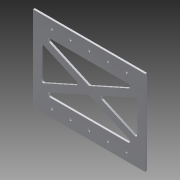
# Autodesk Inventor part: cross_structural_plate(csp)
Saved by Autodesk Inventor 2015 (Build 190159000, 159)
## iProperties
Created: 2015-11-03
Part Number: cross_structural_plate(csp)
Material: Aluminum 6061
Document SubType Name: Sheet Metal
Designer: elilitwack
Density: 2.7 g/cm^3
Sheet Metal Rule: Default
Appearance: Aluminum - Flat
Mass: 129.421 g
Surface Area: 365.561 cm^2
Volume: 47.9336 cm^3
Author: elilitwack
Autodesk Inventor part; units mm, degrees
ref_plane "YZ Plane" through (0, 0, 0) normal (1, 0, 0) x (0, 1, 0)
ref_plane "XZ Plane" through (0, 0, 0) normal (0, 1, 0) x (-1, 0, 0)
ref_plane "XY Plane" through (0, 0, 0) normal (0, 0, 1) x (1, 0, 0)
sketch "profile sketch" plane through (0, 0, 0) normal (0, 0, 1) x (1, 0, 0)
  line L0 (0, 0) -> (180.34, 0)
  line L1 (180.34, 0) -> (180.34, 136.5504)
  line L2 (180.34, 136.5504) -> (0, 136.5504)
  line L3 (0, 136.5504) -> (0, 0)
  dimension "d5" = 180.34
  dimension "d6" = 136.5504
  measures "d5" distance of L1.end L2.end
  measures "d6" distance of L0.end L1.end
extrude "Plate1" add sketch "profile sketch" along normal blind 3.048
sketch "rv_hole_sketch" plane through (0, 0, 3.048) normal (0, 0, 1) x (1, 0, 0)
  line L0 (0, 136.5504) -> (0, 0) construction
  line L1 (180.34, 0) -> (180.34, 136.5504) construction
  line L2 (0, 136.5504) -> (180.34, 136.5504) construction
  line L3 (180.34, 0) -> (0, 0) construction
  line L4 (0, 123.8504) -> (30.0567, 123.8504) construction
  line L5 (30.0567, 123.8504) -> (60.1133, 123.8504) construction
  line L6 (60.1133, 123.8504) -> (90.17, 123.8504) construction
  line L7 (90.17, 123.8504) -> (120.2267, 123.8504) construction
  line L8 (120.2267, 123.8504) -> (150.2833, 123.8504) construction
  line L9 (150.2833, 123.8504) -> (180.34, 123.8504) construction
  line L10 (0, 12.7) -> (30.0567, 12.7) construction
  line L11 (30.0567, 12.7) -> (60.1133, 12.7) construction
  line L12 (60.1133, 12.7) -> (90.17, 12.7) construction
  line L13 (90.17, 12.7) -> (120.2267, 12.7) construction
  line L14 (120.2267, 12.7) -> (150.2833, 12.7) construction
  line L15 (150.2833, 12.7) -> (180.34, 12.7) construction
  dimension "d10" = 12.7
  dimension "d11" = 12.7
  constraints: 24 end point, 13 point on line, 10 coincident, 10 collinear, 3 horizontal
  measures "d10" distance between parallel lines of L3 L13
  measures "d11" distance between parallel lines of L2 L6
hole "rv_holes" at (30.0567, 123.8504, 3.048) at (60.1133, 123.8504, 3.048) at (90.17, 123.8504, 3.048) at (120.2267, 123.8504, 3.048) at (150.2833, 123.8504, 3.048) at (150.2833, 12.7, 3.048) at (120.2267, 12.7, 3.048) at (90.17, 12.7, 3.048) at (60.1133, 12.7, 3.048) at (30.0567, 12.7, 3.048) direction (0, 0, -1) diameter 3.5719 depth 3.048 tip angle 118
sketch "cutout_sketch" plane through (0, 0, 3.048) normal (0, 0, 1) x (1, 0, 0)
  line L0 (12.7, 109.3645) -> (90.17, 74.6252)
  line L1 (90.17, 74.6252) -> (167.64, 109.3645)
  line L2 (167.64, 109.3645) -> (12.7, 109.3645)
  line L3 (12.7, 27.1859) -> (90.17, 61.9252)
  line L4 (90.17, 61.9252) -> (167.64, 27.1859)
  line L5 (167.64, 27.1859) -> (12.7, 27.1859)
  circle A0 centre (90.17, 123.8504) radius 1.7859 projected
  circle A1 centre (90.17, 12.7) radius 1.7859 projected
  line L6 (0, 0) -> (0, 136.5504) projected
  line L7 (180.34, 136.5504) -> (180.34, 0) projected
  line L8 (90.17, 74.6252) -> (90.17, 61.9252) construction
  line L9 (12.7, 96.6645) -> (76.0092, 68.2752)
  line L10 (76.0092, 68.2752) -> (12.7, 39.8859)
  line L11 (12.7, 39.8859) -> (12.7, 96.6645)
  line L12 (167.64, 96.6645) -> (104.3308, 68.2752)
  line L13 (104.3308, 68.2752) -> (167.64, 39.8859)
  line L14 (167.64, 39.8859) -> (167.64, 96.6645)
  line L15 (167.64, 109.3645) -> (167.64, 27.1859) construction
  line L16 (12.7, 109.3645) -> (12.7, 27.1859) construction
  dimension "d36" = 12.7
  dimension "d37" = 12.7
  dimension "d38" = 12.7
  dimension "d39" = 12.7
  dimension "d40" = 12.7
  dimension "d41" = 12.7
  dimension "d42" = 12.7
  dimension "d43" = 12.7
  constraints: 30 end point, 6 equal length, 5 parallel, 3 vertical, 2 collinear, 2 horizontal
  measures "d36" distance edge to line of A0 L2
  measures "d37" distance edge to line of A1 L5
  measures "d38" distance of L0.end L3.end
  measures "d39" distance from line of L6 L3.start
  measures "d40" distance from line of L7 L4.end
  measures "d41" distance of L0.start L9.start
  measures "d42" distance of L3.start L10.end
  measures "d43" distance of L1.end L12.start
extrude "Cut2" cut sketch "cutout_sketch" against normal blind 3.048 contours L2 L1 L0 | L3 L4 L5 | L9 L10 L11 | L14 L13 L12
fillet "Corner Round3" radius 3.175 12 edges at (12.7, 109.3645, 1.524) (167.64, 109.3645, 1.524) (90.17, 74.6252, 1.524) (12.7, 39.8859, 1.524) (12.7, 96.6645, 1.524) (76.0092, 68.2752, 1.524) (90.17, 61.9252, 1.524) (12.7, 27.1859, 1.524) (167.64, 27.1859, 1.524) (104.3308, 68.2752, 1.524) (167.64, 96.6645, 1.524) (167.64, 39.8859, 1.524)
equation "\"d5\" = bh_length"
equation "\"d6\" = bp_height"
equation "\"d10\" = 0.5 * cb_outer_diameter"
equation "\"d11\" = 0.5 * cb_outer_diameter"
equation "\"d12\" = rv_hole_diameter"
equation "\"d17\" = Thickness"
equation "\"d36\" = cmp_mounting_margins"
equation "\"d37\" = cmp_mounting_margins"
equation "\"d38\" = cmp_mounting_margins"
equation "\"d39\" = cmp_mounting_margins"
equation "\"d40\" = cmp_mounting_margins"
equation "\"d41\" = cmp_mounting_margins"
equation "\"d42\" = cmp_mounting_margins"
equation "\"d43\" = cmp_mounting_margins"
equation "\"d44\" = Thickness"
equation "\"d46\" = spd_fillet_size"
equation "\"BendRadius\" = Thickness"
equation "\"BendReliefWidth\" = Thickness"
equation "\"BendReliefDepth\" = 0.5 * Thickness"
equation "\"CornerReliefSize\" = 4 * Thickness"
equation "\"MinimumRemnant\" = 2 * Thickness"
equation "\"TransitionRadius\" = BendRadius"
equation "\"JacobiRadiusSize\" = BendRadius"
equation "\"GapSize\" = Thickness"
equation "\"bh_width\" = 87.63"
equation "\"bh_length\" = 180.34"
equation "\"bh_height\" = bp_height - cb_outer_diameter"
equation "\"bh_metal_width\" = 1.5875"
equation "\"cpn_diameter\" = 69.85"
equation "\"cpn_length\" = 311.15"
equation "\"cmp_foot_seperation_long\" = 139.954"
equation "\"cmp_foot_seperation_short\" = 36.068"
equation "\"cmp_mounting_margins\" = 12.7"
equation "\"cmp_foot_bolt_diameter\" = 6.35"
equation "\"spd_fillet_size\" = 3.175"
equation "\"bp_height\" = gb_mh_seperation + st_outer_diameter"
equation "\"bp_tensioner_width\" = 6.35"
equation "\"bp_tensioner_height\" = 50.8"
equation "\"bp_tensioner_wood_mount_from_tensioner_top\" = 12.7"
equation "\"bp_tensioner_wood_mount_diameter\" = 6.35"
equation "\"cb_outer_diameter\" = 25.4"
equation "\"cb_wall_thickness\" = 1.5875"
equation "\"cb_length\" = 457.2"
equation "\"pdb_mounting_holes_short\" = 104.394"
equation "\"cb_pdb_low_mount_offset\" = 16.0782"
equation "\"pdb_mounting_holes_long\" = 182.2704"
equation "\"pdb_ziptie_hole_diameter\" = 6.35"
equation "\"gb_mh_seperation\" = 111.1504"
equation "\"gb_mh_diameter\" = 6.35"
equation "\"gb_axle_from_edge\" = 38.1"
equation "\"gb_width\" = 127"
equation "\"gb_bearing_diameter\" = 28.575"
equation "\"gb_to_bottom_of_side_assembly\" = 4.7752"
equation "\"ncbt_rivet_row_length\" = 114.3"
equation "\"rv_hole_diameter\" = 3.57187"
equation "\"st_outer_diameter\" = 25.4"
equation "\"st_wall_thickness\" = 1.5875"
equation "\"st_length\" = 685.8"
equation "\"st_gbmh_from_center\" = 55.5752"
equation "\"st_cutout_depth_right\" = 203.2"
equation "\"st_cutout_depth_left\" = 203.2"
equation "\"st_rivet_distance\" = 19.05"
equation "\"so_inner_diameter\" = 7.62"
equation "\"so_wall_thickness\" = 5.08"
equation "\"so_length\" = 40.64"
equation "\"twb_width\" = st_outer_diameter"
equation "\"twb_length\" = bp_tensioner_width + 2 * twb_margin_on_each_side"
equation "\"twb_height\" = 2 * bp_tensioner_wood_mount_diameter + bp_tensioner_height + 2 * bp_tensioner_wood_mount_from_tensioner_top + twb_margin_on_each_side"
equation "\"twb_margin_on_each_side\" = 6.35"
equation "\"twb_tensioner_from_edge\" = -0.5 * bp_tensioner_height + 0.5 * twb_height"
equation "\"tb_rivet_row_length\" = 127"
equation "\"bp_thickness\" = 3.048"
equation "\"bp_width\" = 76.2"
equation "\"bp_axle_height\" = 45.1612"
equation "\"magic_axle_offset\" = 2.286"
equation "\"bp_tensioner_from_bottom\" = 38.1"
equation "\"bp_tensioner_from_side\" = 25.4"
equation "\"d7\" = BendRadius"
equation "\"bh_alternate_height\" = 25.4"
equation "\"bh_alternate_width\" = 81.28"
equation "\"tb_metal_thickness\" = 3.048"
equation "\"tb_hm_mounting_slot_length\" = 40.64"
equation "\"gb_mh_seperation_alt\" = 111.125"
equation "\"gb_axle_from_edge_alt\" = 43.1546"
equation "\"bp_axle_height_alt\" = 50.2158"
equation "\"Thickness\" = 3.048"
body "Solid1"
